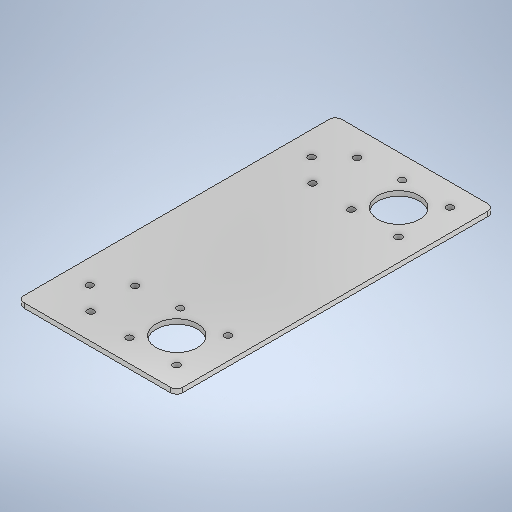
# Autodesk Inventor part: body_bottom_frame
Saved by Autodesk Inventor 2026.1 (Build 301233000, 233)
## iProperties
Created: 2025-08-01
Part Number: body_bottom_frame
Material: Aluminum 6061-AHC
Document SubType Name: Sheet Metal
Designer: chris
Density: 2.7 g/cm^3
Sheet Metal Rule: Default_mm
Appearance: Aluminum - Dark
Flat Pattern Width: 5 cm
Flat Pattern Length: 10 cm
Flat Pattern Area: 50 cm^2
Sheet Metal Width: 50.000 mm
Sheet Metal Length: 100.000 mm
Sheet Metal Area: 5000.000 mm^2
Author: chris
Autodesk Inventor part; units mm, degrees
ref_plane "YZ Plane" through (0, 0, 0) normal (1, 0, 0) x (0, 1, 0)
ref_plane "XZ Plane" through (0, 0, 0) normal (0, 1, 0) x (-1, 0, 0)
ref_plane "XY Plane" through (0, 0, 0) normal (0, 0, 1) x (1, 0, 0)
sketch "Sketch1" plane through (0, 0, 0) normal (0, 1, 0) x (-1, 0, 0)
  line L0 (-25, 50) -> (25, 50)
  line L1 (25, 50) -> (25, -50)
  line L2 (25, -50) -> (-25, -50)
  line L3 (-25, -50) -> (-25, 50)
  line L4 (-25, 50) -> (25, -50) construction
  line L5 (25, 50) -> (-25, -50) construction
  point P0 (0, 0)
  dimension "d0" = 50
  dimension "d1" = 100
  measures "d0" distance of L1.end L2.end
  measures "d1" distance of L0.end L1.end
extrude "Plate1" add sketch "Sketch1" along normal blind 1.5
fillet "Fillet1" radius 2 4 edges at (25, 0.75, 50) (25, 0.75, -50) (-25, 0.75, -50) (-25, 0.75, 50)
sketch "Sketch5" plane through (0, 1.5, 0) normal (0, 1, 0) x (1, 0, 0)
  circle A0 centre (-17.42, -34.93) radius 0.7835 projected
  circle A1 centre (-10.12, -41.93) radius 0.7835 projected
  circle A2 centre (-10.12, -27.93) radius 0.7835 projected
  circle A3 centre (3.1, -42.93) radius 0.7835 projected
  circle A4 centre (3.1, -26.93) radius 0.7835 projected
  line L0 (-18.82, -28.86) -> (-18.82, -41) projected
  line L1 (-18.82, -28.86) -> (-18.1, -28.86) projected
  arc A5 (-18.1, -28.86) -> (-16.1, -26.86) centre (-18.1, -26.86) ccw projected
  line L2 (-16.1, -26.86) -> (-16.1, -26.14) projected
  line L3 (16, -26.14) -> (-16.1, -26.14) projected
  line L4 (16, -26.14) -> (16, -26.86) projected
  arc A6 (16, -26.86) -> (18, -28.86) centre (18, -26.86) ccw projected
  line L5 (18, -28.86) -> (18.72, -28.86) projected
  line L6 (18.72, -41) -> (18.72, -28.86) projected
  line L7 (18.72, -41) -> (18, -41) projected
  arc A7 (18, -41) -> (16, -43) centre (18, -43) ccw projected
  line L8 (16, -43) -> (16, -43.72) projected
  line L9 (-16.1, -43.72) -> (16, -43.72) projected
  line L10 (-16.1, -43.72) -> (-16.1, -43) projected
  arc A8 (-16.1, -43) -> (-18.1, -41) centre (-18.1, -43) ccw projected
  line L11 (-18.1, -41) -> (-18.82, -41) projected
  circle A9 centre (10, -34.93) radius 6.4 projected
  circle A10 centre (-17.42, 34.93) radius 0.7835 projected
  circle A11 centre (-10.12, 27.93) radius 0.7835 projected
  circle A12 centre (-10.12, 41.93) radius 0.7835 projected
  circle A13 centre (3.1, 26.93) radius 0.7835 projected
  circle A14 centre (3.1, 42.93) radius 0.7835 projected
  line L12 (-18.82, 41) -> (-18.82, 28.86) projected
  line L13 (-18.82, 41) -> (-18.1, 41) projected
  arc A15 (-18.1, 41) -> (-16.1, 43) centre (-18.1, 43) ccw projected
  line L14 (-16.1, 43) -> (-16.1, 43.72) projected
  line L15 (16, 43.72) -> (-16.1, 43.72) projected
  line L16 (16, 43.72) -> (16, 43) projected
  arc A16 (16, 43) -> (18, 41) centre (18, 43) ccw projected
  line L17 (18, 41) -> (18.72, 41) projected
  line L18 (18.72, 28.86) -> (18.72, 41) projected
  line L19 (18.72, 28.86) -> (18, 28.86) projected
  arc A17 (18, 28.86) -> (16, 26.86) centre (18, 26.86) ccw projected
  line L20 (16, 26.86) -> (16, 26.14) projected
  line L21 (-16.1, 26.14) -> (16, 26.14) projected
  line L22 (-16.1, 26.14) -> (-16.1, 26.86) projected
  arc A18 (-16.1, 26.86) -> (-18.1, 28.86) centre (-18.1, 26.86) ccw projected
  line L23 (-18.1, 28.86) -> (-18.82, 28.86) projected
  circle A19 centre (10, 34.93) radius 6.4 projected
  point P0 (0, 0)
hole "Hole3" at (-17.42, 1.5, 34.93) at (-10.12, 1.5, 27.93) at (-10.12, 1.5, 41.93) at (3.1, 1.5, 42.93) at (3.1, 1.5, 26.93) at (18, 1.5, 26.86) at (18, 1.5, 43) at (18, 1.5, -26.86) at (18, 1.5, -43) at (3.1, 1.5, -42.93) at (3.1, 1.5, -26.93) at (-10.12, 1.5, -41.93) at (-10.12, 1.5, -27.93) at (-17.42, 1.5, -34.93) direction (0, -1, 0) diameter 2.1 depth 1.5 tip angle 118
sketch "Sketch6" plane through (0, 1.5, 0) normal (0, 1, 0) x (1, 0, 0)
  circle A0 centre (-17.42, -34.93) radius 0.7835 projected
  circle A1 centre (-10.12, -41.93) radius 0.7835 projected
  circle A2 centre (-10.12, -27.93) radius 0.7835 projected
  circle A3 centre (3.1, -42.93) radius 0.7835 projected
  circle A4 centre (3.1, -26.93) radius 0.7835 projected
  line L0 (-18.82, -28.86) -> (-18.82, -41) projected
  line L1 (-18.82, -28.86) -> (-18.1, -28.86) projected
  arc A5 (-18.1, -28.86) -> (-16.1, -26.86) centre (-18.1, -26.86) ccw projected
  line L2 (-16.1, -26.86) -> (-16.1, -26.14) projected
  line L3 (16, -26.14) -> (-16.1, -26.14) projected
  line L4 (16, -26.14) -> (16, -26.86) projected
  arc A6 (16, -26.86) -> (18, -28.86) centre (18, -26.86) ccw projected
  line L5 (18, -28.86) -> (18.72, -28.86) projected
  line L6 (18.72, -41) -> (18.72, -28.86) projected
  line L7 (18.72, -41) -> (18, -41) projected
  arc A7 (18, -41) -> (16, -43) centre (18, -43) ccw projected
  line L8 (16, -43) -> (16, -43.72) projected
  line L9 (-16.1, -43.72) -> (16, -43.72) projected
  line L10 (-16.1, -43.72) -> (-16.1, -43) projected
  arc A8 (-16.1, -43) -> (-18.1, -41) centre (-18.1, -43) ccw projected
  line L11 (-18.1, -41) -> (-18.82, -41) projected
  circle A9 centre (10, -34.93) radius 6.4 projected
  circle A10 centre (-17.42, 34.93) radius 0.7835 projected
  circle A11 centre (-10.12, 27.93) radius 0.7835 projected
  circle A12 centre (-10.12, 41.93) radius 0.7835 projected
  circle A13 centre (3.1, 26.93) radius 0.7835 projected
  circle A14 centre (3.1, 42.93) radius 0.7835 projected
  line L12 (-18.82, 41) -> (-18.82, 28.86) projected
  line L13 (-18.82, 41) -> (-18.1, 41) projected
  arc A15 (-18.1, 41) -> (-16.1, 43) centre (-18.1, 43) ccw projected
  line L14 (-16.1, 43) -> (-16.1, 43.72) projected
  line L15 (16, 43.72) -> (-16.1, 43.72) projected
  line L16 (16, 43.72) -> (16, 43) projected
  arc A16 (16, 43) -> (18, 41) centre (18, 43) ccw projected
  line L17 (18, 41) -> (18.72, 41) projected
  line L18 (18.72, 28.86) -> (18.72, 41) projected
  line L19 (18.72, 28.86) -> (18, 28.86) projected
  arc A17 (18, 28.86) -> (16, 26.86) centre (18, 26.86) ccw projected
  line L20 (16, 26.86) -> (16, 26.14) projected
  line L21 (-16.1, 26.14) -> (16, 26.14) projected
  line L22 (-16.1, 26.14) -> (-16.1, 26.86) projected
  arc A18 (-16.1, 26.86) -> (-18.1, 28.86) centre (-18.1, 26.86) ccw projected
  line L23 (-18.1, 28.86) -> (-18.82, 28.86) projected
  circle A19 centre (10, 34.93) radius 6.4 projected
  circle A20 centre (10, -34.93) radius 6.5
  circle A21 centre (10, 34.93) radius 6.5
  point P0 (0, 0)
  dimension "d27" = 13
  dimension "d28" = 13
  constraints: 2 centre point, 2 coincident
  measures "d27" diameter of A20
  measures "d28" diameter of A21
extrude "Cut2" cut sketch "Sketch6" against normal blind 1.5 contours A9 | A19 | A20 | A21
equation "\"d25\" = Thickness"
equation "\"d29\" = Thickness"
equation "\"d2\" = Thickness"
equation "\"BendReliefWidth\" = Thickness"
equation "\"BendReliefDepth\" = 0.5 * Thickness"
equation "\"CornerReliefSize\" = 4 * Thickness"
equation "\"MinimumRemnant\" = 2 * Thickness"
equation "\"TransitionRadius\" = BendRadius"
equation "\"JacobiRadiusSize\" = BendRadius"
equation "\"GapSize\" = Thickness"
equation "\"Thickness\" = 1.5"
equation "\"BendRadius\" = 0.31"
body "Solid1"
